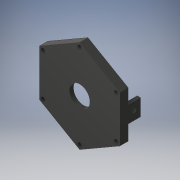
# Autodesk Inventor part: TA01
Saved by Autodesk Inventor 2017 (Build 210142000, 142)
## iProperties
Created: 2018-10-09
Part Number: TA01
Material: ABS Plastic
Document SubType Name: Modeling
Designer: Zach
Density: 1.06 g/cm^3
Appearance: Smooth - Black
Author: Zach
Autodesk Inventor part; units mm, degrees
ref_plane "YZ Plane" through (0, 0, 0) normal (1, 0, 0) x (0, 1, 0)
ref_plane "XZ Plane" through (0, 0, 0) normal (0, 1, 0) x (-1, 0, 0)
ref_plane "XY Plane" through (0, 0, 0) normal (0, 0, 1) x (1, 0, 0)
sketch "Sketch1" plane through (0, 0, 0) normal (0, 0, 1) x (1, 0, 0)
  circle A0 centre (0, 0) radius 12.5
  circle A1 centre (-30, 0) radius 3
  circle A2 centre (-15, -25.9808) radius 3
  circle A3 centre (15, -25.9808) radius 3
  circle A4 centre (30, 0) radius 3
  circle A5 centre (15, 25.9808) radius 3
  circle A6 centre (-15, 25.9808) radius 3
  line L0 (0, 56) -> (48.4974, 28)
  line L1 (48.4974, 28) -> (48.4974, -28)
  line L2 (48.4974, -28) -> (0, -56)
  line L3 (0, -56) -> (-48.4974, -28)
  line L4 (-48.4974, -28) -> (-48.4974, 28)
  line L5 (-48.4974, 28) -> (0, 56)
  point P0 (48.4974, 0)
  dimension "d0" = 25
  dimension "d2" = 6
  dimension "d6" = 360
  dimension "d15" = 30
  dimension "d33" = 112
  constraints: 12 end point, 7 centre point, 2 coincident, 2 horizontal alignment, 1 midpoint, 26 other
  measures "d0" diameter of A0
  measures "d2" diameter of A1
  measures "d15" distance of point (0, 0) A1.centre
  measures "d33" distance of L2.end L0.start
extrude "Extrusion1" add sketch "Sketch1" along normal blind 10 contours A1 | A2 | A3 | A4 | A5 | A6 | L0 L1 L2 L3 L4 L5
sketch "Sketch7" plane through (0, 0, 10) normal (0, 0, 1) x (1, 0, 0)
  circle A0 centre (0, 51) radius 2.5
  line L0 (48.4974, 28) -> (0, 56) projected
  circle A1 centre (-44.1673, 25.5) radius 2.5
  circle A2 centre (-44.1673, -25.5) radius 2.5
  circle A3 centre (0, -51) radius 2.5
  circle A4 centre (44.1673, -25.5) radius 2.5
  circle A5 centre (44.1673, 25.5) radius 2.5
  point P0 (0, 0)
  dimension "d42" = 5
  dimension "d43" = 5
  dimension "d46" = 360
  constraints: 6 centre point, 1 vertical alignment, 13 other
  measures "d42" diameter of A0
  measures "d43" distance of L0.end A0.centre
extrude "Extrusion6" cut sketch "Sketch7" against normal through all
sketch "Sketch9" plane through (0, 0, 0) normal (0, 0, -1) x (-1, 0, 0)
  circle A0 centre (0, 0) radius 25
  dimension "d56" = 50
  constraints: 1 centre point, 1 coincident
  measures "d56" diameter of A0
extrude "Extrusion8" cut sketch "Sketch9" against normal blind 5
sketch "Sketch12" plane through (0, 0, 10) normal (0, 0, 1) x (1, 0, 0)
  line L0 (-48.4974, 28) -> (-48.4974, -28) projected
  line L1 (-44.4974, 10) -> (-48.4974, 10)
  line L2 (-48.4974, 10) -> (-48.4974, -10)
  line L3 (-48.4974, -10) -> (-44.4974, -10)
  line L4 (-44.4974, -10) -> (-44.4974, 10)
  line L5 (44.4974, 10) -> (48.4974, 10)
  line L6 (48.4974, 10) -> (48.4974, -10)
  line L7 (48.4974, -10) -> (44.4974, -10)
  line L8 (44.4974, -10) -> (44.4974, 10)
  line L9 (48.4974, -28) -> (48.4974, 28) projected
  point P0 (0, 0)
  point P1 (-48.4974, 0)
  point P2 (48.4974, 0)
  dimension "d72" = 4
  dimension "d73" = 4
  dimension "d74" = 20
  dimension "d75" = 20
  constraints: 16 end point, 4 midpoint, 4 parallel, 2 horizontal, 2 perpendicular
  measures "d72" distance of L1.start L1.end
  measures "d73" distance of L5.start L5.end
  measures "d74" distance of L1.end L2.end
  measures "d75" distance of L5.end L6.end
extrude "Extrusion11" add sketch "Sketch12" against normal blind 25
sketch "Sketch13" plane through (-48.4974, -10, 10) normal (-1, 0, 0) x (0, 0, 1)
  line L0 (-10, 20) -> (-10, 0) projected
  line L1 (-10, 20) -> (-25, 20) projected
  line L2 (-25, 0) -> (-25, 20) projected
  line L3 (-10, 0) -> (-25, 0) projected
  circle A0 centre (-17.5, 10) radius 2.5
  point P0 (-10, 10)
  point P1 (-17.5, 20)
  point P2 (-25, 10)
  dimension "d78" = 5
  constraints: 2 midpoint, 1 centre point, 1 horizontal alignment, 1 vertical alignment
  measures "d78" diameter of A0
extrude "Extrusion12" cut sketch "Sketch13" against normal through all contours A0
body "Solid1"
